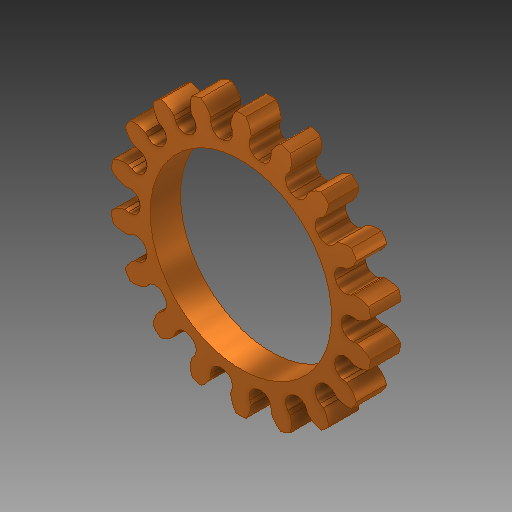
# Autodesk Inventor part: IRGear
Saved by Autodesk Inventor 2017 (Build 210142000, 142)
## iProperties
Created: 2017-02-15
Part Number: IRGear
Material: Gold
Document SubType Name: Modeling
Designer: Moonlight.Admin
Density: 19.3 g/cm^3
Appearance: Metal 1600F Hot
Author: Moonlight.Admin
Autodesk Inventor part; units mm, degrees
ref_plane "YZ Plane" through (0, 0, 0) normal (1, 0, 0) x (0, 1, 0)
ref_plane "XZ Plane" through (0, 0, 0) normal (0, 1, 0) x (-1, 0, 0)
ref_plane "XY Plane" through (0, 0, 0) normal (0, 0, 1) x (1, 0, 0)
derived "CombinedHousingV2.ipt"
sketch "IR Distance" plane through (0, 0, 0) normal (0, 0, 1) x (1, 0, 0)
  line L0 (36.2, -29.125) -> (36.2, -50.625) construction
  line L1 (56.625, -24.13) -> (30.125, -24.13) construction
  circle A0 centre (12.7, 42) radius 9
  circle A1 centre (12.7, 42) radius 12.5
  circle A2 centre (-7.3, 42) radius 5
  circle A3 centre (32.7, 42) radius 5
  circle A4 centre (-7.3, 42) radius 1.905
  circle A5 centre (32.7, 42) radius 1.905
  circle A6 centre (-7.3, 42) radius 3.4925
  circle A7 centre (32.7, 42) radius 3.4925
  point P0 (0, 0)
sketch "Sketch2" plane through (0, 0, 0) normal (0, 0, 1) x (1, 0, 0)
  circle A0 centre (12.7, 42) radius 9 projected
  arc A1 (12.2, 29.0428) -> (13.2, 29.0428) centre (12.7, 32.0008) ccw
  arc A2 (13.2, 29.0428) -> (13.7, 31.0428) centre (10.9766, 30.6611) ccw
  line L0 (12.2, 29.0428) -> (13.2, 29.0428) construction
  arc A3 (11.7, 31.0428) -> (12.2, 29.0428) centre (14.4234, 30.6611) ccw
  line L1 (11.7, 31.0428) -> (13.7, 31.0428) construction
  arc A4 (11.7, 31.0428) -> (9.7097, 31.1816) centre (10.7097, 31.1816) ccw
  arc A5 (15.6903, 31.1816) -> (13.7, 31.0428) centre (14.6903, 31.1816) ccw
  line L2 (9.7097, 31.1816) -> (9.7097, 28.5428)
  line L3 (9.7097, 28.5428) -> (15.6903, 28.5428)
  line L4 (15.6903, 28.5428) -> (15.6903, 31.1816)
  line L5 (12.7, 50.2535) -> (12.7, 38.8443) construction
  circle A6 centre (12.7, 42) radius 10 construction
  circle A7 centre (12.7, 42) radius 12.9992
  point P0 (0, 0)
  point P1 (12.7, 31.0428)
  point P2 (12.7, 29.0428)
  dimension "d1" = 3
  dimension "d2" = 2
  dimension "d3" = 0.5
  dimension "d4" = 1
  dimension "d5" = 2
  dimension "d6" = 2.75
  dimension "d8" = 1
  dimension "d9" = 1
  constraints: 13 end point, 10 point on circle, 7 centre point, 6 tangent, 3 point on line, 2 coincident, 2 equal radius, 2 midpoint, 2 parallel, 1 perpendicular, 1 vertical
  measures "d1" radius of A1
  measures "d2" distance of L1.end L1.start
  measures "d3" distance between parallel lines of L3 L0
  measures "d4" radius of A4
  measures "d5" distance between parallel lines of L0 L1
  measures "d6" radius of A3
  measures "d8" distance of L0.end L0.start
  measures "d9" radial gap between concentric circles of A6 A0
extrude "Extrusion1" add sketch "Sketch2" along normal blind 3 contours A3 A4 L2 A7 L4 A5 A2 A1 | A1 A7 L2 A4 A3 | A1 A2 A5 L4 A7
extrude "Extrusion2" cut sketch "Sketch2" along normal blind 3 contours A1 A7 L2 A4 A3 | A7 L4 L3 L2 | A1 A2 A5 L4 A7
pattern_circular "Circular Pattern1" count 18 over 360 about axis through (12.7, 42, 0) along (0, 0, 1) of "Extrusion2"
body "Solid1"
